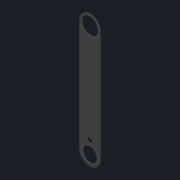
# Autodesk Inventor part: link2-plate2
Saved by Autodesk Inventor 2021 (Build 250183000, 183)
## iProperties
Created: 2021-07-15
Part Number: link2-plate2
Material: CFRP
Document SubType Name: Sheet Metal
Designer: yuta0
Density: 1.43 g/cm^3
Sheet Metal Rule: Default
Appearance: カーボンファイバー
Mass: 100.539 g
Surface Area: 741.112 cm^2
Volume: 70.3069 cm^3
購入先: カーボン
在庫数: 0.0
Author: yuta0
Autodesk Inventor part; units mm, degrees
ref_plane "YZ Plane" through (0, 0, 0) normal (1, 0, 0) x (0, 1, 0)
ref_plane "XZ Plane" through (0, 0, 0) normal (0, 1, 0) x (-1, 0, 0)
ref_plane "XY Plane" through (0, 0, 0) normal (0, 0, 1) x (1, 0, 0)
sketch "スケッチ1" plane through (0, 0, 0) normal (0, 0, 1) x (1, 0, 0)
  circle A0 centre (0, 0) radius 40.5
  circle A1 centre (0, 440) radius 40.5
  line L0 (-40.5, 0) -> (-40.5, 440)
  line L1 (40.5, 440) -> (40.5, 0)
  dimension "d0" = 81
  dimension "d1" = 81
  dimension "d2" = 440
  measures "d0" diameter of A0
  measures "d1" diameter of A1
  measures "d2" distance of A0.centre A1.centre
extrude "プレート1" add sketch "スケッチ1" along normal blind 2
sketch "スケッチ4" plane through (0, 0, 0) normal (0, 0, -1) x (-1, 0, 0)
  circle A0 centre (0, 0) radius 28
  dimension "d28" = 56
  constraints: 1 centre point, 1 coincident
  measures "d28" diameter of A0
extrude "押し出し1" cut sketch "スケッチ4" against normal blind 10
sketch "スケッチ5" plane through (0, 0, 0) normal (0, 0, -1) x (-1, 0, 0)
  circle A0 centre (0, 0) radius 32
  point P0 (0, 32)
  point P1 (-27.7128, 16)
  point P2 (-27.7128, -16)
  point P3 (0, -32)
  point P4 (27.7128, -16)
  point P5 (27.7128, 16)
  dimension "d31" = 64
  dimension "d34" = 360
  constraints: 1 coincident, 1 vertical alignment, 9 other
hole "穴3" at (0, 32, 0) at (27.7128, 16, 0) at (27.7128, -16, 0) at (0, -32, 0) at (-27.7128, -16, 0) at (-27.7128, 16, 0) direction (0, 0, 1) diameter 4.3 end through all clearance for "Flat Head Machine Screw" size "M4" standard "Ansi Metric M Profile"
sketch "スケッチ6" plane through (0, 0, 2) normal (0, 0, 1) x (1, 0, 0)
  arc A0 (40.5, 440) -> (-40.5, 440) centre (0, 440) ccw projected
  circle A1 centre (0, 440) radius 32.55
  point P0 (0, 0)
  dimension "d43" = 65.1
  constraints: 1 centre point, 1 coincident
  measures "d43" diameter of A1
extrude "押し出し2" cut sketch "スケッチ6" against normal blind 10
sketch "スケッチ9" plane through (0, 0, 2) normal (0, 0, 1) x (1, 0, 0)
  arc A0 (40.5, 440) -> (-40.5, 440) centre (0, 440) ccw projected
  circle A1 centre (0, 440) radius 36.5
  point P0 (0, 0)
  point P1 (0, 476.5)
  point P2 (-31.6099, 458.25)
  point P3 (-31.6099, 421.75)
  point P4 (0, 403.5)
  point P5 (31.6099, 421.75)
  point P6 (31.6099, 458.25)
  dimension "d58" = 73
  dimension "d61" = 360
  constraints: 1 coincident, 1 vertical alignment, 9 other
hole "穴5" at (0, 476.5, 2) at (-31.6099, 458.25, 2) at (-31.6099, 421.75, 2) at (0, 403.5, 2) at (31.6099, 421.75, 2) at (31.6099, 458.25, 2) direction (0, 0, -1) diameter 3.2 end through all clearance for "Socket Head Cap Screw" size "M3" standard "Ansi Metric M Profile"
sketch "スケッチ16" plane through (0, 0, 2) normal (0, 0, 1) x (1, 0, 0)
  circle A0 centre (0, 355.2097) radius 4
  arc A1 (40.5, 440) -> (-40.5, 440) centre (0, 440) ccw projected
  circle A2 centre (0, 440) radius 25
  line L0 (-23.4923, 431.4495) -> (4.1883, 355.3977)
  line L1 (0, 603.9) -> (0, -147.9) projected
  point P0 (0, 0)
  dimension "d154" = 50
  dimension "d135" = 8
  dimension "d136" = 0
  dimension "d137" = 160
  constraints: 2 end point, 1 centre point, 1 coincident, 1 tangent, 4 other
  measures "d135" diameter of A0
  measures "d136" horizontal distance of A1.centre A0.centre
  measures "d137" angle of L0 L1
hole "穴11" at (0, 355.2097, 2) direction (0, 0, -1) diameter 4.5 end through all clearance for "Flat Head Machine Screw" size "M4" standard "Ansi Metric M Profile"
sketch "スケッチ17" plane through (0, 0, 2) normal (0, 0, 1) x (1, 0, 0)
  circle A0 centre (0, 0) radius 44
  point P0 (-4, 72)
  dimension "d145" = 88
  dimension "d177" = 72
  dimension "d178" = 4
  constraints: 1 centre point, 1 coincident
  measures "d145" diameter of A0
  measures "d177" vertical distance of point (0, 0) point (-4, 72)
  measures "d178" horizontal distance of point (0, 0) point (-4, 72)
hole "穴12" at (-4, 72, 2) direction (0, 0, -1) diameter 4.3 end through all clearance for "Flat Head Machine Screw" size "M4" standard "Ansi Metric M Profile"
sketch "スケッチ18" plane through (0, 0, 0) normal (0, 0, -1) x (-1, 0, 0)
  line L0 (-9, 41) -> (9, 41)
  line L1 (9, 41) -> (9, 56)
  line L2 (9, 56) -> (-9, 56)
  line L3 (-9, 56) -> (-9, 41)
  line L4 (-9, 41) -> (9, 56) construction
  line L5 (9, 41) -> (-9, 56) construction
  arc A0 (40.5, 440) -> (-40.5, 440) centre (0, 440) ccw projected
  point P0 (0, 0)
  point P1 (0, 48.5)
  point P2 (0, 48.5)
  dimension "d157" = 18
  dimension "d158" = 15
  dimension "d183" = 41
  constraints: 12 end point, 3 midpoint, 2 parallel, 1 horizontal, 1 perpendicular, 1 vertical alignment
  measures "d157" distance of L2.end L1.end
  measures "d158" distance of L1.end L0.end
  measures "d183" distance from line of point (0, 0) L0
extrude "押し出し4" cut sketch "スケッチ18" against normal blind 10
fillet "コーナーR2" radius 2 4 edges at (-9, 56, 1) (9, 56, 1) (9, 41, 1) (-9, 41, 1)
sketch "スケッチ19" plane through (0, 0, 2) normal (0, 0, 1) x (1, 0, 0)
  line L0 (21, 72) -> (-4, 72) construction
  line L1 (21, 69.85) -> (-4, 69.85)
  line L2 (-4, 74.15) -> (21, 74.15)
  arc A0 (21, 69.85) -> (21, 74.15) centre (21, 72) ccw
  arc A1 (-4, 74.15) -> (-4, 69.85) centre (-4, 72) ccw
  circle A2 centre (-4, 72) radius 2.15 projected
  point P0 (0, 0)
  point P1 (8.5, 72)
  dimension "d182" = 21
  constraints: 8 end point, 5 tangent, 4 point on circle, 2 centre point, 1 coincident, 1 horizontal alignment, 1 midpoint, 1 parallel
  measures "d182" horizontal distance of point (0, 0) L0.start
extrude "押し出し5" cut sketch "スケッチ19" against normal blind 10
sketch "スケッチ20" plane through (0, 0, 0) normal (0, 0, -1) x (-1, 0, 0)
  point P0 (0, 0)
  point P1 (0, 220)
  dimension "d167" = 220
  measures "d167" distance of point (0, 0) point (0, 220)
hole "穴13" at (0, 220, 0) direction (0, 0, 1) diameter 4.3 end through all clearance for "Flat Head Machine Screw" size "M4" standard "Ansi Metric M Profile"
equation "\"d41\" = Thickness"
equation "\"d68\" = Thickness"
equation "\"d143\" = Thickness"
equation "\"d152\" = Thickness"
equation "\"d173\" = Thickness"
equation "\"d3\" = Thickness"
equation "\"BendRadius\" = Thickness"
equation "\"BendReliefWidth\" = Thickness"
equation "\"BendReliefDepth\" = 0.5 * Thickness"
equation "\"CornerReliefSize\" = 4 * Thickness"
equation "\"MinimumRemnant\" = 2 * Thickness"
equation "\"TransitionRadius\" = BendRadius"
equation "\"JacobiRadiusSize\" = Thickness"
equation "\"GapSize\" = Thickness"
equation "\"Thickness\" = 2"
